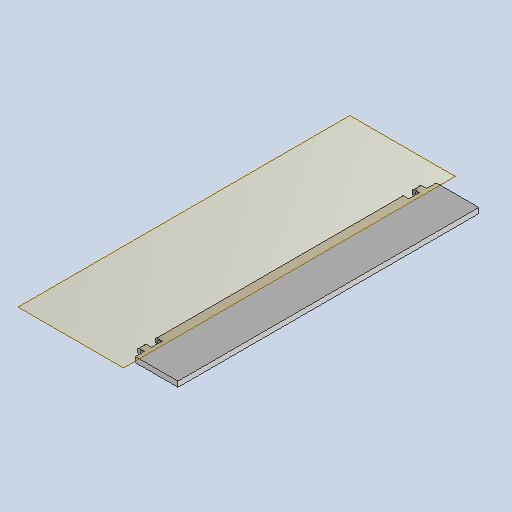
# Autodesk Inventor part: pokrow2
Saved by Autodesk Inventor 2024 (Build 280153000, 153)
## iProperties
Created: 2023-09-16
Part Number: pokrow2
Material: Generic
Document SubType Name: Modeling
Designer: jebes windows
Density: 1 g/cm^3
Appearance: Default
Author: jebes windows
Autodesk Inventor part; units mm, degrees
ref_plane "YZ Plane" through (0, 0, 0) normal (1, 0, 0) x (0, 1, 0)
ref_plane "XZ Plane" through (0, 0, 0) normal (0, 1, 0) x (-1, 0, 0)
ref_plane "XY Plane" through (0, 0, 0) normal (0, 0, 1) x (1, 0, 0)
ref_plane "Work Plane1" through (0, 0, 0) normal (0, 0, 1) x (1, 0, 0)
sketch "Sketch1" plane through (0, 0, 0) normal (0, 0, 1) x (1, 0, 0)
  line L0 (29, 75) -> (29, 70) projected
  line L1 (25, 75) -> (29, 75) projected
  line L2 (25, 75) -> (25, 80) projected
  line L3 (25, 80) -> (29, 80) projected
  line L4 (29, 85) -> (29, 80) projected
  line L5 (-25, 85) -> (29, 85) projected
  line L6 (-25, 85) -> (-25, -85) projected
  line L7 (-25, -85) -> (29, -85) projected
  line L8 (29, -80) -> (29, -85) projected
  line L9 (25, -80) -> (29, -80) projected
  line L10 (25, -80) -> (25, -75) projected
  line L11 (25, -75) -> (29, -75) projected
  line L12 (29, -70) -> (29, -75) projected
  line L13 (25, -70) -> (29, -70) projected
  line L14 (25, -70) -> (25, 70) projected
  line L15 (25, 70) -> (29, 70) projected
  line L16 (25.5, -75.5) -> (25.5, -79.5)
  line L17 (25.5, -79.5) -> (29.5, -79.5)
  line L18 (29.5, -79.5) -> (29.5, -85.5)
  line L19 (29.5, -85.5) -> (-25.5, -85.5)
  line L20 (-25.5, -85.5) -> (-25.5, 85.5)
  line L21 (-25.5, 85.5) -> (29.5, 85.5)
  line L22 (29.5, 85.5) -> (29.5, 79.5)
  line L23 (29.5, 79.5) -> (25.5, 79.5)
  line L24 (25.5, 79.5) -> (25.5, 75.5)
  line L25 (25.5, 75.5) -> (29.5, 75.5)
  line L26 (29.5, 75.5) -> (29.5, 69.5)
  line L27 (29.5, 69.5) -> (25.5, 69.5)
  line L28 (25.5, 69.5) -> (25.5, -69.5)
  line L29 (25.5, -69.5) -> (29.5, -69.5)
  line L30 (29.5, -69.5) -> (29.5, -75.5)
  line L31 (29.5, -75.5) -> (25.5, -75.5)
  line L32 (29.5, -84.5715) -> (53.5, -84.5715)
  line L33 (53.5, -84.5715) -> (53.5, 85)
  line L34 (53.5, 85) -> (29.5, 85)
  point P0 (0, 0)
  point P1 (29, -82.5)
  point P2 (29, 82.5)
  dimension "d0" = 0.5
  dimension "d1" = 24
  dimension "d2" = 2.0715
  dimension "d3" = 2.5
  constraints: 38 end point, 2 midpoint, 2 perpendicular, 2 point on line, 1 horizontal, 15 other
  measures "d0" distance between parallel lines of L10 L16
  measures "d1" distance of L32.start L32.end
  measures "d2" distance from line of point (29, -82.5) L32
  measures "d3" distance from line of point (29, 82.5) L34
extrude "Extrusion1" add sketch "Sketch1" against normal blind 3 contours L31 L30 L29 L28 L27 L26 L25 L24 L23 L22 L34 L33 L32 L18 L17 L16
sketch "Sketch2" plane through (25.5, 79.5, 0) normal (0, 1, 0) x (1, 0, 0)
  circle A0 centre (2.5, 1.5) radius 1
  line L0 (0, 0) -> (0, 3) projected
  circle A1 centre (2, -6.0738) radius 1 projected
  arc A2 (4.5, -5.5738) -> (3.5, -4.5738) centre (3.5, -5.5738) ccw projected
  line L1 (-0.5, -4.5738) -> (3.5, -4.5738) projected
  line L2 (-0.5, 20.4262) -> (-0.5, -4.5738) projected
  line L3 (-0.5, 25.4262) -> (-0.5, 20.4262) projected
  line L4 (-0.5, 25.4262) -> (-180.5, 25.4262) projected
  line L5 (-180.5, 25.4262) -> (-180.5, 20.4262) projected
  line L6 (-50.5, 20.4262) -> (-180.5, 20.4262) projected
  line L7 (-50.5, 20.4262) -> (-50.5, -7.5738) projected
  line L8 (-50.5, -7.5738) -> (3.5, -7.5738) projected
  arc A3 (3.5, -7.5738) -> (4.5, -6.5738) centre (3.5, -6.5738) ccw projected
  line L9 (4.5, -6.5738) -> (4.5, -5.5738) projected
  line L10 (0, 3) -> (4, 3) projected
  point P0 (-25.5, 0)
  point P1 (0, 1.5)
  dimension "d6" = 2
  dimension "d7" = 2.5
  dimension "d8" = 1.5
  constraints: 1 centre point, 1 midpoint
  measures "d6" diameter of A0
  measures "d7" distance of point (0, 1.5) A0.centre
  measures "d8" distance from line of L10 A0.centre
extrude "Extrusion2" cut sketch "Sketch2" against normal through all contours A0
fillet "Fillet1" radius 1 6 edges at (25.5, 0, 0) (25.5, 0, -3) (25.5, -77.5, 0) (25.5, -77.5, -3) (25.5, 77.5, 0) (25.5, 77.5, -3)
body "Solid1"
